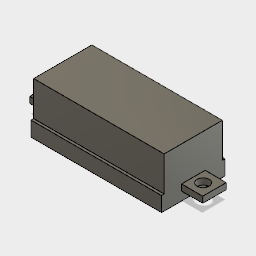
potenceBatteryPack (Autodesk Fusion 360 archive; units mm, degrees)
design "7segDisplay"
Autodesk Fusion 360 part; units mm, degrees
sketch "Sketch1" plane through (0, 0, 0) normal (0, 1, 0) x (1, 0, 0)
  line L0 (11.3, 5.05) -> (-11.3, 5.05)
  line L1 (-11.3, 5.05) -> (-11.3, -5.05)
  line L2 (-11.3, -5.05) -> (11.3, -5.05)
  line L3 (11.3, -5.05) -> (11.3, 5.05)
  line L4 (11.3, 5.05) -> (-11.3, -5.05) construction
  line L5 (-11.3, 5.05) -> (11.3, -5.05) construction
  dimension "d1" = 22.6
  dimension "d2" = 10.1
  constraint perpendicular L0 L1
  constraint parallel L0 L2
  constraint parallel L1 L3
  constraint horizontal L0
  constraint coincident L4
  constraint coincident L5
extrude "Extrude1" add sketch "Sketch1" along normal blind 6
sketch "Sketch2" plane through (0, 0, 0) normal (0, -1, 0) x (1, 0, 0)
  line L0 (11.3, -5.05) -> (11.3, 5.05)
  line L1 (11.3, 5.05) -> (-11.3, 5.05)
  line L2 (-11.3, 5.05) -> (-11.3, -5.05)
  line L3 (-11.3, -5.05) -> (11.3, -5.05)
  line L4 (11.3, -5.5) -> (-11.3, -5.5)
  line L5 (-11.3, 5.5) -> (11.3, 5.5)
  line L6 (11.3, -5.5) -> (-11.3, 5.5) construction
  line L7 (-11.3, -5.5) -> (11.3, 5.5) construction
  line L8 (-11.3, -2.04) -> (-14.97, -2.04)
  line L9 (-14.97, -2.04) -> (-14.97, 2.04)
  line L10 (-14.97, 2.04) -> (-11.3, 2.04)
  line L11 (-14.97, 0) -> (0, 0) construction
  line L12 (0, 5.5) -> (0, -5.5) construction
  line L13 (11.3, -2.04) -> (14.97, -2.04)
  line L14 (14.97, -2.04) -> (14.97, 2.04)
  line L15 (14.97, 2.04) -> (11.3, 2.04)
  line L16 (-11.3, 2.04) -> (-11.3, 5.5)
  line L17 (-11.3, -5.5) -> (-11.3, -5.05)
  line L18 (-11.3, -2.04) -> (-11.3, 0)
  line L19 (-11.3, -5.05) -> (-11.3, -2.04)
  line L20 (11.3, 5.5) -> (11.3, 2.04)
  line L21 (11.3, -2.04) -> (11.3, -5.5)
  line L22 (11.3, 2.04) -> (11.3, -2.04)
  dimension "d5" = 22.6
  dimension "d6" = 11
  dimension "d7" = 4.08
  dimension "d8" = 3.67
  constraint perpendicular L4 L17
  constraint parallel L4 L5
  constraint parallel L17 L20
  constraint horizontal L4
  constraint coincident L6
  constraint coincident L7
  constraint horizontal L8
  constraint vertical L9
  constraint horizontal L10
  constraint coincident L17
  constraint coincident L9
  constraint horizontal L11
  constraint midpoint L5
  constraint midpoint L4
  constraint horizontal L13
  constraint vertical L14
  constraint horizontal L15
  constraint coincident L20
  constraint coincident L11
extrude "Extrude2" add sketch "Sketch2" along normal blind 1.08
sketch "Sketch3" plane through (0, -1.08, 0) normal (0, -1, 0) x (1, 0, 0)
  line L0 (14.97, -2.04) -> (14.97, 2.04)
  line L1 (14.97, 2.04) -> (11.3, 2.04)
  line L2 (11.3, 2.04) -> (11.3, 5.5)
  line L3 (11.3, 5.5) -> (-11.3, 5.5)
  line L4 (-11.3, 5.5) -> (-11.3, 2.04)
  line L5 (-11.3, 2.04) -> (-14.97, 2.04)
  line L6 (-14.97, 2.04) -> (-14.97, -2.04)
  line L7 (-14.97, -2.04) -> (-11.3, -2.04)
  line L8 (-11.3, -2.04) -> (-11.3, -5.5)
  line L9 (-11.3, -5.5) -> (11.3, -5.5)
  line L10 (11.3, -5.5) -> (11.3, -2.04)
  line L11 (11.3, -2.04) -> (14.97, -2.04)
  circle A0 centre (-13, 0) radius 1.05
  circle A1 centre (13, 0) radius 1.05
  line L12 (0, 5.5) -> (0, -5.5) construction
  line L13 (-13, 0) -> (13, 0) construction
  dimension "d11" = 2.1
  dimension "d12" = 13
  constraint midpoint L3
  constraint midpoint L9
  constraint coincident L13
  measures "d11" diameter of A0
  measures "d12" distance of L12
extrude "Extrude3" cut sketch "Sketch3" against normal up to surface (1.08 mm away) contours A0 | A1
sketch "Sketch4" plane through (0, -1.08, 0) normal (0, -1, 0) x (1, 0, 0)
  circle A0 centre (13, 0) radius 1.05
  circle A1 centre (-13, 0) radius 1.05
  line L0 (14.97, -2.04) -> (14.97, 2.04)
  line L1 (14.97, 2.04) -> (11.3, 2.04)
  line L2 (11.3, 2.04) -> (11.3, 5.5)
  line L3 (11.3, 5.5) -> (-11.3, 5.5)
  line L4 (-11.3, 5.5) -> (-11.3, 2.04)
  line L5 (-11.3, 2.04) -> (-14.97, 2.04)
  line L6 (-14.97, 2.04) -> (-14.97, -2.04)
  line L7 (-14.97, -2.04) -> (-11.3, -2.04)
  line L8 (-11.3, -2.04) -> (-11.3, -5.5)
  line L9 (-11.3, -5.5) -> (11.3, -5.5)
  line L10 (11.3, -5.5) -> (11.3, -2.04)
  line L11 (11.3, -2.04) -> (14.97, -2.04)
  line L12 (-11.3, 5.5) -> (11.3, 5.5)
  line L13 (11.3, 5.5) -> (11.3, -5.5)
  line L14 (11.3, -5.5) -> (-11.3, -5.5)
  line L15 (-11.3, -5.5) -> (-11.3, 5.5)
extrude "Extrude4" add sketch "Sketch4" along normal blind 1.5 contours L2 L3 L4 L8 L9 L10 L12 L13 L14 L15

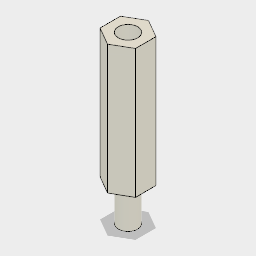
design "colonnette"
Autodesk Fusion 360 part; units mm, degrees
sketch "Sketch1" plane through (0, 0, 0) normal (0, 1, 0) x (1, 0, 0)
  line L0 (2.75, 1.5877) -> (0, 3.1754)
  line L1 (0, 3.1754) -> (-2.75, 1.5877)
  line L2 (-2.75, 1.5877) -> (-2.75, -1.5877)
  line L3 (-2.75, -1.5877) -> (0, -3.1754)
  line L4 (0, -3.1754) -> (2.75, -1.5877)
  line L5 (2.75, -1.5877) -> (2.75, 1.5877)
  dimension "d1" = 5.5
  constraint vertical L5
  measures "d1" distance of L2 L5
extrude "Extrude1" add sketch "Sketch1" along normal blind 20
sketch "Sketch2" plane through (0, 20, 0) normal (0, 1, 0) x (-1, 0, 0)
  line L0 (-2.75, 1.5877) -> (-2.75, -1.5877)
  line L1 (-2.75, -1.5877) -> (0, -3.1754)
  line L2 (0, -3.1754) -> (2.75, -1.5877)
  line L3 (2.75, -1.5877) -> (2.75, 1.5877)
  line L4 (2.75, 1.5877) -> (0, 3.1754)
  line L5 (0, 3.1754) -> (-2.75, 1.5877)
  circle A0 centre (0, 0) radius 1.5
  dimension "d4" = 3
  measures "d4" diameter of A0
extrude "Extrude2" cut sketch "Sketch2" against normal blind 17 contours A0
sketch "Sketch3" plane through (0, 0, 0) normal (0, -1, 0) x (1, 0, 0)
  line L0 (2.75, -1.5877) -> (2.75, 1.5877)
  line L1 (2.75, 1.5877) -> (0, 3.1754)
  line L2 (0, 3.1754) -> (-2.75, 1.5877)
  line L3 (-2.75, 1.5877) -> (-2.75, -1.5877)
  line L4 (-2.75, -1.5877) -> (0, -3.1754)
  line L5 (0, -3.1754) -> (2.75, -1.5877)
  circle A0 centre (0, 0) radius 1.5
  constraint coincident A0
extrude "Extrude3" add sketch "Sketch3" along normal blind 5.7 contours A0

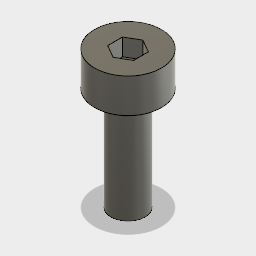
design "visHC2x6"
Autodesk Fusion 360 part; units mm, degrees
sketch "Sketch1" plane through (0, 0, 0) normal (0, 1, 0) x (1, 0, 0)
  circle A0 centre (0, 0) radius 1.95
  dimension "d1" = 3.9
  measures "d1" diameter of A0
extrude "Extrude1" add sketch "Sketch1" along normal blind 2
sketch "Sketch2" plane through (0, 0, 0) normal (0, -1, 0) x (1, 0, 0)
  circle A0 centre (0, 0) radius 1.95
  circle A1 centre (0, 0) radius 1
  dimension "d4" = 2
  constraint concentric A0 A1
  measures "d4" diameter of A1
extrude "Extrude2" add sketch "Sketch2" along normal blind 6 contours A1
sketch "Sketch3" plane through (0, 2, 0) normal (0, 1, 0) x (-1, 0, 0)
  circle A0 centre (0, 0) radius 1.95
  line L0 (-0.75, -0.433) -> (0, -0.866)
  line L1 (0, -0.866) -> (0.75, -0.433)
  line L2 (0.75, -0.433) -> (0.75, 0.433)
  line L3 (0.75, 0.433) -> (0, 0.866)
  line L4 (0, 0.866) -> (-0.75, 0.433)
  line L5 (-0.75, 0.433) -> (-0.75, -0.433)
  constraint vertical L5
extrude "Extrude3" cut sketch "Sketch3" against normal blind 1 contours L0 L1 L2 L3 L4 L5
